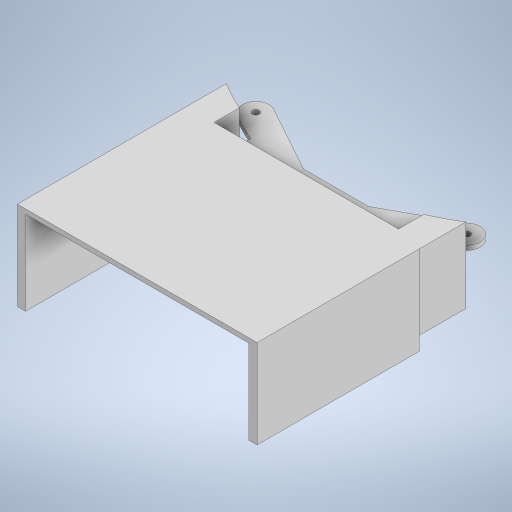
# Autodesk Inventor part: tampa_principal_v2
Saved by Autodesk Inventor 2024.3 (Build 283343000, 343)
## iProperties
Created: 2025-02-24
Part Number: tampa_principal_v2
Material: Genérico
Document SubType Name: Modeling
Designer: lostv
Density: 1 g/cm^3
Appearance: Padrão
Author: lostv
Autodesk Inventor part; units mm, degrees
ref_plane "YZ Plane" through (0, 0, 0) normal (1, 0, 0) x (0, 1, 0)
ref_plane "XZ Plane" through (0, 0, 0) normal (0, 1, 0) x (-1, 0, 0)
ref_plane "XY Plane" through (0, 0, 0) normal (0, 0, 1) x (1, 0, 0)
sketch "Esboço1" plane through (0, 0, 0) normal (0, 1, 0) x (-1, 0, 0)
  line L0 (-64.0727, 52.888) -> (39.938, 52.888)
  line L1 (39.938, 52.888) -> (39.938, -22.879)
  line L2 (-64.0727, -22.8617) -> (-64.0727, 52.888)
  line L3 (24.938, -35.9271) -> (-49.07, -35.9082)
  line L4 (24.938, -35.9271) -> (24.938, -22.982)
  line L5 (-49.07, -35.9082) -> (-49.07, -22.982)
  line L6 (27.938, -33.9512) -> (27.938, -22.982)
  line L7 (-52.07, -22.982) -> (-52.07, -33.9417)
  line L8 (-64.0727, -22.8617) -> (-64.0727, -40.2203)
  line L9 (-60.562, -22.879) -> (-60.5704, -38.1726) construction
  line L10 (39.938, -22.879) -> (39.938, -40.2377)
  circle A0 centre (-57.062, -28.879) radius 1.75
  circle A1 centre (32.938, -28.879) radius 1.75
  circle A2 centre (33.72, -46.8489) radius 1.5
  circle A3 centre (20.938, -31.0333) radius 1.75
  line L11 (24.938, -35.9271) -> (24.938, -22.982)
  circle A4 centre (-45.062, -31.0333) radius 1.75
  line L12 (-49.07, -35.9271) -> (-49.07, -22.982)
  circle A5 centre (-57.8544, -46.8314) radius 1.5
  circle A6 centre (-57.8544, -46.8314) radius 5.8468
  line L13 (-54.0723, -51.2901) -> (-26.1853, -35.9201)
  circle A7 centre (33.7303, -46.8314) radius 5.8468
  line L14 (29.9483, -51.2901) -> (2.0612, -35.9201)
  ellipse E0 centre (-12.062, -134.482) end of major axis (91.4576, -134.482) minor radius 109.0206 (-49.07, -32.666) -> (-64.0727, -40.2203) ccw
  ellipse E1 centre (-12.062, -134.482) end of major axis (91.438, -134.482) minor radius 109 (39.938, -40.2377) -> (24.938, -32.6849) ccw
  ellipse E2 centre (-12.062, -134.482) end of major axis (-12.062, -240.5307) minor radius 100.3503 (-49.07, -35.9082) -> (-60.5723, -41.6475) ccw
  ellipse E3 centre (-12.062, -134.482) end of major axis (-12.062, -240.482) minor radius 100.5 (36.438, -41.6421) -> (24.938, -35.9271) ccw
  line L15 (-26.1853, -35.9201) -> (-26.1743, -35.914)
  line L16 (2.0612, -35.9201) -> (2.0633, -35.9213)
  line L17 (36.438, -41.6421) -> (36.4459, -41.6535)
  line L18 (-60.5723, -41.6475) -> (-60.5868, -41.6623)
  line L19 (29.938, -22.9847) -> (29.938, -22.982)
  line L20 (36.4326, -22.982) -> (36.4326, 52.888)
  line L21 (-60.5566, -22.982) -> (-60.5566, 52.888)
  line L22 (39.938, 50.388) -> (-64.0727, 50.388)
  line L23 (39.938, -19.982) -> (36.4326, -19.982)
  line L24 (39.938, -22.982) -> (-64.0727, -22.982)
  line L25 (-60.5566, -19.982) -> (-64.0727, -19.982)
  point P0 (0, 0)
  point P1 (-13.31, 23.8291)
  point P2 (-12.062, -22.982)
  point P3 (63.9356, 48.927)
  point P4 (59.9356, 42.927)
  point P5 (-12.062, -28.482)
  point P6 (-12.062, -22.982)
  point P7 (-52.07, -35.7207)
  point P8 (-52.07, -28.4725)
  point P9 (-49.07, -29.4451)
  point P10 (-52.07, -30.1013)
  point P11 (24.938, -32.6849)
  point P12 (-49.07, -32.666)
  point P13 (24.938, -29.4545)
  point P14 (-49.07, -29.4545)
  point P15 (36.4326, 50.388)
  point P16 (-60.5566, 50.388)
  point P17 (38.1853, -19.982)
  point P18 (-12.062, -22.982)
  point P19 (-60.5566, -22.982)
  point P20 (-52.07, -33.9323)
  dimension "d2" = 3
  dimension "d3" = 3
  dimension "d6" = 66
  dimension "d16" = 3.5054
  dimension "d17" = 3.516
  dimension "d18" = 2.5
  dimension "d20" = 104.0106
  dimension "d27" = 12.9451
  dimension "d28" = 88.8152
  dimension "d29" = 3
  constraints: 52 end point, 20 point on line, 8 centre point, 5 perpendicular, 4 midpoint, 4 point on circle, 4 vertical, 3 horizontal, 2 coincident, 2 parallel, 1 collinear, 18 other
  measures "d2" horizontal distance of point (-49.07, -29.445) point (-52.07, -30.101)
  measures "d3" distance from line of point (24.938, -32.685) L6
  measures "d6" distance of A3.centre A4.centre
  measures "d16" distance between parallel lines of L20 L1
  measures "d17" distance between parallel lines of L2 L21
  measures "d18" distance between parallel lines of L0 L22
  measures "d20" distance between parallel lines of L2 L1
  measures "d27" distance of L11.end L3.start
  measures "d28" distance from line of L0 L11.start
  measures "d29" distance between parallel lines of L24 L23
extrude "Extrusão1" add sketch "Esboço1" against normal blind 2 contours L22 L20 L24 L21
extrude "Extrusão2" add sketch "Esboço1" against normal blind 38.5 contours L22 L21 L25 L2 | L22 L1 L23 L20
extrude "Extrusão3" add sketch "Esboço1" against normal blind 32.5 contours L25 L21 L24 L8 L2 | L23 L1 L10 L24 L20 | L24 L7 E0 L8 | L24 L10 E1 L6 | A0 | A1
extrude "Extrusão4" add sketch "Esboço1" against normal blind 13 contours L24 L4 L3 L5 | L3 L15 L13 A6 L18 E2 | E3 L17 A7 L14 L3 | A6 | A7
extrude "Extrusão5" cut sketch "Esboço1" against normal blind 11 contours L24 L4 L3 L5 | L3 L15 L13 A6 L18 E2 | E3 L17 A7 L14 L3 | A6 | A7 | A2 | A5
